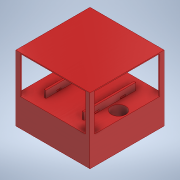
# Autodesk Inventor part: CajaBoya
Saved by Autodesk Inventor 2020 (Build 240168000, 168)
## iProperties
Created: 2021-10-16
Part Number: CajaBoya
Material: Genérico
Document SubType Name: Modeling
Designer: DANIEL
Density: 1 g/cm^3
Appearance: Rojo
Author: DANIEL
Autodesk Inventor part; units mm, degrees
ref_plane "YZ Plane" through (0, 0, 0) normal (1, 0, 0) x (0, 1, 0)
ref_plane "XZ Plane" through (0, 0, 0) normal (0, 1, 0) x (-1, 0, 0)
ref_plane "XY Plane" through (0, 0, 0) normal (0, 0, 1) x (1, 0, 0)
sketch "Boceto1" plane through (0, 0, 0) normal (0, 1, 0) x (-1, 0, 0)
  line L0 (200, 200) -> (-200, 200)
  line L1 (-200, 200) -> (-200, -200)
  line L2 (-200, -200) -> (200, -200)
  line L3 (200, -200) -> (200, 200)
  point P0 (0, 0)
  dimension "d0" = 400
  dimension "L" = 400
  dimension "d2" = 200
  dimension "d3" = 200
  constraints: 8 end point, 2 parallel, 1 horizontal, 1 perpendicular
  measures "d0" distance between parallel lines of L1 L3
  measures "L" distance between parallel lines of L2 L0
  measures "d2" distance from line of L1 point (0, 0)
  measures "d3" distance from line of point (0, 0) L0
extrude "Extrusión1" add sketch "Boceto1" along normal blind 150
sketch "Boceto3" plane through (0, 150, 0) normal (0, 1, 0) x (1, 0, 0)
  circle A0 centre (0, -121) radius 39
  line L0 (200, 200) -> (-200, 200) projected
  line L1 (-200, -200) -> (200, -200) projected
  point P0 (0, 0)
  dimension "D" = 78
  dimension "d27" = 79
  constraints: 1 centre point
  measures "D" diameter of A0
  measures "d27" distance from line of L1 A0.centre
extrude "Extrusión2" [suppressed]
ref_plane "Plano de trabajo1" through (0, 0, 200) normal (1, 0, 0) x (0, 0, -1)
ref_plane "Plano de trabajo2" through (-200, 0, 0) normal (0, 0, 1) x (1, 0, 0)
sketch "Boceto4" plane through (0, 150, 0) normal (0, 1, 0) x (1, 0, 0)
  line L0 (-97.5, 140) -> (-97.5, -140)
  line L1 (97.5, 140) -> (97.5, -140)
  line L2 (200, 200) -> (-200, 200) projected
  circle A0 centre (0, -121) radius 39 projected
  line L3 (-200, -200) -> (200, -200) projected
  line L4 (-97.5, -140) -> (-107.5, -140)
  line L5 (-107.5, -140) -> (-107.5, 140)
  line L6 (-107.5, 140) -> (-97.5, 140)
  line L7 (-97.5, 140) -> (-97.5, -140)
  line L8 (97.5, -140) -> (107.5, -140)
  line L9 (107.5, -140) -> (107.5, 140)
  line L10 (107.5, 140) -> (97.5, 140)
  line L11 (97.5, 140) -> (97.5, -140)
  point P0 (0, 0)
  dimension "Lriel" = 280
  dimension "d13" = 60
  dimension "d14" = 280
  dimension "d15" = 60
  dimension "d19" = 10
  dimension "d20" = 280
  dimension "d21" = 97.5
  dimension "d22" = 10
  dimension "d23" = 280
  dimension "d24" = 97.5
  constraints: 20 end point, 4 parallel, 2 horizontal, 2 perpendicular, 2 vertical
  measures "Lriel" distance of L0.start L0.end
  measures "d13" distance from line of L2 L0.start
  measures "d14" distance of L1.start L1.end
  measures "d15" distance from line of L2 L1.start
  measures "d19" distance of L5.end L6.end
  measures "d20" distance of L4.end L5.end
  measures "d21" distance from line of point (0, 0) L0
  measures "d22" distance of L10.end L9.end
  measures "d23" distance of L9.end L8.end
  measures "d24" distance from line of point (0, 0) L1
extrude "Extrusión3" add sketch "Boceto4" along normal blind 38 contours L0 L4 L5 L6 | L10 L9 L8 L1
sketch "Boceto5" plane through (0, 150, 0) normal (0, 1, 0) x (1, 0, 0)
  line L0 (-200, 200) -> (-200, -200) projected
  line L1 (-200, 200) -> (-200, 175)
  line L2 (-200, 175.482) -> (-195, 175.482)
  line L3 (-195, 175.482) -> (-195, 195.482)
  line L4 (-195, 195.482) -> (-175, 195.482)
  line L5 (-175, 195.482) -> (-175, 200)
  line L6 (200, 200) -> (-200, 200) projected
  line L7 (-200, 200) -> (-175, 200)
  line L8 (-200, -200) -> (-200, -175)
  line L9 (-200, -175) -> (-195, -175)
  line L10 (-195, -175) -> (-195, -195)
  line L11 (-195, -195) -> (-175, -195)
  line L12 (-175, -195) -> (-175, -200)
  line L13 (-200, -200) -> (200, -200) projected
  line L14 (-175, -200) -> (-200, -200)
  line L15 (200, -200) -> (200, 200) projected
  line L16 (200, -200) -> (200, -175)
  line L17 (200, -175) -> (195, -175)
  line L18 (195, -175) -> (195, -195)
  line L19 (195, -195) -> (175, -195)
  line L20 (175, -195) -> (175, -200)
  line L21 (200, -200) -> (175, -200)
  line L22 (200, 200) -> (200, 175)
  line L23 (200, 175) -> (195, 175)
  line L24 (195, 175) -> (195, 195)
  line L25 (195, 195) -> (175, 195)
  line L26 (175, 195) -> (175, 200)
  line L27 (200, 200) -> (175, 200)
  point P0 (0, 0)
  dimension "d28" = 25
  dimension "d29" = 5
  dimension "d30" = 20
  dimension "d31" = 20
  dimension "d32" = 25
  dimension "d33" = 5
  dimension "d34" = 20
  dimension "d35" = 20
  dimension "d36" = 25
  dimension "d37" = 5
  dimension "d38" = 20
  dimension "d39" = 20
  dimension "d40" = 25
  dimension "d41" = 5
  dimension "d42" = 20
  dimension "d43" = 20
  constraints: 48 end point, 16 perpendicular, 9 point on line, 2 collinear, 2 horizontal
  measures "d28" distance of L0.start L1.end
  measures "d29" distance of L2.start L2.end
  measures "d30" distance of L2.end L3.end
  measures "d31" distance of L3.end L4.end
  measures "d32" distance of L0.end L8.end
  measures "d33" distance of L8.end L9.end
  measures "d34" distance of L9.end L10.end
  measures "d35" distance of L10.end L11.end
  measures "d36" distance of L13.end L16.end
  measures "d37" distance of L16.end L17.end
  measures "d38" distance of L17.end L18.end
  measures "d39" distance of L18.end L19.end
  measures "d40" distance of L6.start L22.end
  measures "d41" distance of L22.end L23.end
  measures "d42" distance of L23.end L24.end
  measures "d43" distance of L24.end L25.end
extrude "Extrusión4" add sketch "Boceto5" along normal blind 200 contours L6 L5 L4 L3 L2 L0 | L6 L15 L23 L24 L25 L26 | L9 L10 L11 L12 L13 L0 | L15 L13 L20 L19 L18 L17
sketch "Boceto6" plane through (0, 350, 0) normal (0, 1, 0) x (1, 0, 0)
  line L0 (-200, 200) -> (-200, -200) projected
  line L1 (-200, -200) -> (200, -200)
  line L2 (200, -200) -> (200, 200)
  line L3 (200, 200) -> (-200, 200)
  line L4 (-200, 200) -> (-200, -200)
  point P0 (0, 0)
  constraints: 8 end point, 2 parallel, 1 horizontal, 1 perpendicular
extrude "Extrusión5" add sketch "Boceto6" along normal blind 5
sketch "Boceto7" plane through (0, 150, 0) normal (0, 1, 0) x (1, 0, 0)
  line L0 (-200, 200) -> (-200, -200) projected
  line L1 (200, 200) -> (-200, 200) projected
  line L2 (200, -200) -> (200, 200) projected
  line L3 (-200, -200) -> (200, -200) projected
  circle A0 centre (154, 0) radius 39
  point P0 (0, 0)
  dimension "d48" = 78
  dimension "d49" = 200
  dimension "d50" = 46
  constraints: 1 centre point
  measures "d48" diameter of A0
  measures "d49" distance from line of L1 A0.centre
  measures "d50" distance from line of L2 A0.centre
extrude "Extrusión6" cut sketch "Boceto7" against normal blind 200.5 contours A0
sketch "Boceto8" plane through (107.5, 150, 140) normal (1, 0, 0) x (0, 0, -1)
  line L0 (61.75, 6.3333) -> (78.25, 6.3333) construction
  line L1 (61.75, 10.3333) -> (78.25, 10.3333)
  line L2 (78.25, 2.3333) -> (61.75, 2.3333)
  arc A0 (61.75, 10.3333) -> (61.75, 2.3333) centre (61.75, 6.3333) ccw
  arc A1 (78.25, 2.3333) -> (78.25, 10.3333) centre (78.25, 6.3333) ccw
  line L3 (0, 38) -> (280, 38) projected
  line L4 (0, 0) -> (0, 38) projected
  line L5 (198.75, 6.3333) -> (221.25, 6.3333) construction
  line L6 (315.482, 0) -> (-35, 0) projected
  line L7 (198.75, 10.3333) -> (221.25, 10.3333)
  line L8 (221.25, 2.3333) -> (198.75, 2.3333)
  arc A2 (198.75, 10.3333) -> (198.75, 2.3333) centre (198.75, 6.3333) ccw
  arc A3 (221.25, 2.3333) -> (221.25, 10.3333) centre (221.25, 6.3333) ccw
  line L9 (280, 0) -> (280, 38) projected
  point P0 (140, -150)
  point P1 (70, 6.3333)
  point P2 (210, 6.3333)
  dimension "d53" = 31.6667
  dimension "d54" = 70
  dimension "d55" = 4
  dimension "d56" = 31.6667
  dimension "d57" = 4
  dimension "d58" = 70
  constraints: 16 end point, 8 point on circle, 8 tangent, 4 centre point, 3 parallel, 2 midpoint, 1 horizontal
  measures "d53" distance between parallel lines of L3 L0
  measures "d54" distance from line of L4 point (70, 6.333)
  measures "d55" distance from line of L1 point (70, 6.333)
  measures "d56" distance between parallel lines of L3 L5
  measures "d57" distance from line of L7 point (210, 6.333)
  measures "d58" distance from line of point (210, 6.333) L9
extrude "Extrusión7" cut sketch "Boceto8" against normal blind 251.25 contours L1 A1 L2 A0 | L7 A3 L8 A2
equation "\"d0\" = L"
equation "\"d2\" = 0.5 * L"
equation "\"d3\" = 0.5 * L"
equation "\"d14\" = Lriel"
